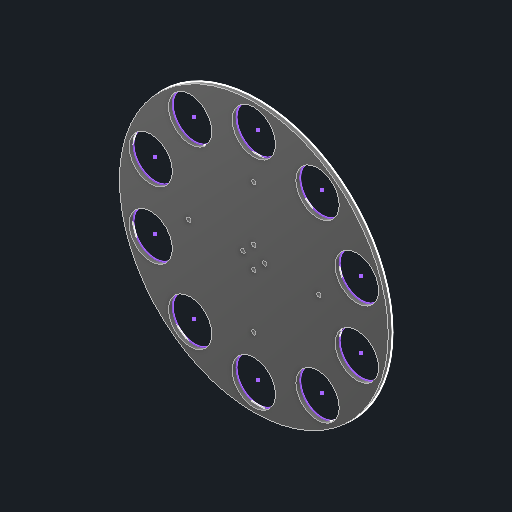
# Autodesk Inventor part: Part2
Saved by Autodesk Inventor 2027.1 (Build 311270010, 270A)
## iProperties
Created: 2026-09-28
Part Number: Part2
Material: Acetal Resin, Black
Document SubType Name: Modeling
Designer: daniel
Density: 1.425 g/cm^3
Appearance: Smooth - Black
Mass: 397.644 g
Surface Area: 1245.44 cm^2
Volume: 279.048 cm^3
Author: daniel
Autodesk Inventor part; units mm, degrees
ref_plane "YZ Plane" through (0, 0, 0) normal (1, 0, 0) x (0, 1, 0)
ref_plane "XZ Plane" through (0, 0, 0) normal (0, 1, 0) x (-1, 0, 0)
ref_plane "XY Plane" through (0, 0, 0) normal (0, 0, 1) x (1, 0, 0)
sketch "Sketch1" plane through (0, 0, 0) normal (0, 0, 1) x (1, 0, 0)
  circle A0 centre (0, 0) radius 150
  circle A1 centre (0, 0) radius 100
  circle A2 centre (0, -125) radius 25
  circle A3 centre (73.4732, -101.1271) radius 25
  circle A4 centre (118.8821, -38.6271) radius 25
  circle A5 centre (118.8821, 38.6271) radius 25
  circle A6 centre (73.4732, 101.1271) radius 25
  circle A7 centre (0, 125) radius 25
  circle A8 centre (-73.4732, 101.1271) radius 25
  circle A9 centre (-118.8821, 38.6271) radius 25
  circle A10 centre (-118.8821, -38.6271) radius 25
  circle A11 centre (-73.4732, -101.1271) radius 25
  circle A12 centre (0, 0) radius 50
  circle A13 centre (0, 0) radius 155
  circle A14 centre (0, 0) radius 12.5
  circle A15 centre (12.5, 0) radius 2.5
  circle A16 centre (0, -12.5) radius 2.5
  circle A17 centre (-12.5, 0) radius 2.5
  circle A18 centre (0, 12.5) radius 2.5
  circle A19 centre (0, 0) radius 7
  circle A20 centre (0, 7) radius 1.6
  circle A21 centre (7, 0) radius 1.6
  circle A22 centre (0, -7) radius 1.6
  circle A23 centre (-7, 0) radius 1.6
  circle A24 centre (0, 0) radius 75
  circle A25 centre (-75, 0) radius 2.5
  circle A26 centre (0, -75) radius 2.5
  circle A27 centre (75, 0) radius 2.5
  circle A28 centre (0, 75) radius 2.5
  dimension "d36" = 150
  dimension "d0" = 300
  dimension "d1" = 200
  dimension "d2" = 50
  dimension "d5" = 360
  dimension "d7" = 100
  dimension "d13" = 310
  dimension "d17" = 25
  dimension "d18" = 5
  dimension "d19" = 5
  dimension "d20" = 5
  dimension "d21" = 5
  dimension "d29" = 14
  dimension "d30" = 3.2
  dimension "d31" = 3.2
  dimension "d32" = 3.2
  dimension "d33" = 3.2
  dimension "d37" = 5
  dimension "d40" = 360
  constraints: 28 centre point, 8 point on circle, 7 coincident, 1 horizontal alignment, 1 tangent, 32 other
  measures "d0" diameter of A0
  measures "d1" diameter of A1
  measures "d2" diameter of A2
  measures "d7" diameter of A12
  measures "d13" diameter of A13
  measures "d17" diameter of A14
  measures "d18" diameter of A15
  measures "d19" diameter of A16
  measures "d20" diameter of A17
  measures "d21" diameter of A18
  measures "d29" diameter of A19
  measures "d30" diameter of A20
  measures "d31" diameter of A21
  measures "d32" diameter of A22
  measures "d33" diameter of A23
  measures "d37" diameter of A25
extrude "Extrusion1" add sketch "Sketch1" along normal blind 5 contours A0 A4 A1 A5 | A5 A1 A6 A0 | A0 A3 A1 A4 | A6 A1 A7 A0 | A1 | A0 A2 A1 A3 | A7 A1 A8 A0 | A0 A11 A1 A2 | A8 A1 A9 A0 | A0 A10 A1 A11 | A9 A1 A10 A0 | A12 | A13 | A15 A14 A16 A17 A18 | A19 A21 | A19 A21 | A21 A19 A22 A23 A20 | A20 A19 | A19 A20 | A22 A19 | A19 A22 | A23 A19 | A19 A23 | A27 A24 A26 A25 A28
equation "\"d0\" = 6 * Product_dia"
equation "\"d1\" = 4 * Product_dia"
equation "\"d2\" = Product_dia"
equation "\"d7\" = 2 * Product_dia"
equation "\"Product_dia\" = 50"
equation "\"GridTotalSize\" = 63"
equation "\"GridBorderThickness\" = 5"
equation "\"GridBorderFillets\" = 7"
equation "\"BaseTotalWidth\" = 652"
equation "\"GridProcutClearance\" = 3"
equation "\"WorkspaceLength\" = 552"
equation "\"AxesBaseFillet\" = 15"
equation "\"WorkspaceWidth\" = 417"
equation "\"ProductTotalHeight\" = 45"
equation "\"VerticalStroke\" = 85"
equation "\"Zaxis\" = 223"
equation "\"WorkspaceHeight\" = 136.5"
equation "\"BaseTotalLength\" = 912"
equation "\"DistanceBetweenGrid\" = 5"
equation "\"CylinderStroke\" = 75"
equation "\"BaseWoodThickness\" = 7"
equation "\"kerf\" = 1.5"
equation "\"Kerf\" = 0.3"
equation "\"RxThickness\" = 1.8"
body "Solid1"
